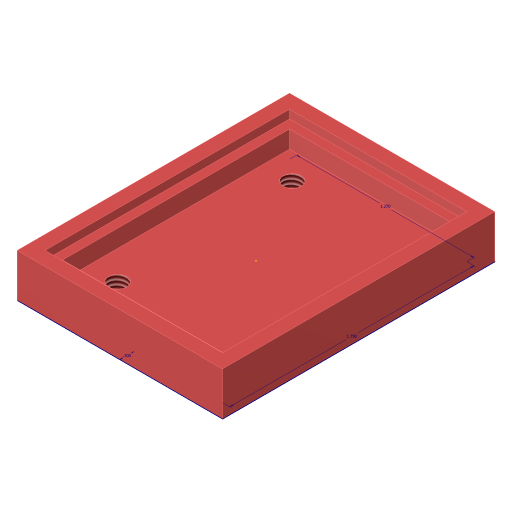
# Autodesk Inventor part: TOF mount
Saved by Autodesk Inventor 2023.4 (Build 274418000, 418)
## iProperties
Created: 2025-02-18
Part Number: TOF mount
Material: ABS Plastic
Document SubType Name: Modeling
Designer: mavericks
Density: 1.06 g/cm^3
Appearance: Smooth - Red
Author: mavericks
Autodesk Inventor part; units mm, degrees
ref_plane "YZ Plane" through (0, 0, 0) normal (1, 0, 0) x (0, 1, 0)
ref_plane "XZ Plane" through (0, 0, 0) normal (0, 1, 0) x (-1, 0, 0)
ref_plane "XY Plane" through (0, 0, 0) normal (0, 0, 1) x (1, 0, 0)
sketch "Sketch2" plane through (0, 0, 0) normal (0, 1, 0) x (-1, 0, 0)
  line L0 (16.129, 22.225) -> (-16.129, 22.225)
  line L1 (-16.129, 22.225) -> (-16.129, -22.225)
  line L2 (-16.129, -22.225) -> (16.129, -22.225)
  line L3 (16.129, -22.225) -> (16.129, 22.225)
  line L4 (16.129, 22.225) -> (-16.129, -22.225) construction
  line L5 (-16.129, 22.225) -> (16.129, -22.225) construction
  line L6 (-18.669, 24.765) -> (18.669, 24.765)
  line L7 (18.669, 24.765) -> (18.669, -24.765)
  line L8 (18.669, -24.765) -> (-18.669, -24.765)
  line L9 (-18.669, -24.765) -> (-18.669, 24.765)
  point P0 (0, 0)
  dimension "d0" = 32.258
  dimension "d1" = 44.45
  dimension "d2" = 2.54
  constraints: 20 end point, 4 parallel, 2 midpoint, 2 perpendicular, 1 horizontal, 3 other
  measures "d0" distance of L2.end L1.end
  measures "d1" distance of L1.end L0.end
  measures "d2" distance between parallel lines of L0 L6
extrude "Extrusion1" add sketch "Sketch2" along normal blind 3.175 contours L3 L2 L1 L0
extrude "Extrusion2" add sketch "Sketch2" along normal blind 7.874
sketch "Sketch3" plane through (0, 3.175, 0) normal (0, 1, 0) x (1, 0, 0)
  line L0 (16.129, 22.225) -> (16.129, -22.225) projected
  line L1 (16.129, -22.225) -> (-16.129, -22.225) projected
  point P0 (0, 0)
  point P1 (-9.271, -15.875)
  point P2 (-9.271, 15.875)
  dimension "d7" = 25.4
  dimension "d8" = 25.4
  dimension "d9" = 6.35
  dimension "d10" = 38.1
  measures "d7" distance from line of L0 point (-9.271, -15.875)
  measures "d8" distance from line of L0 point (-9.271, 15.875)
  measures "d9" distance from line of point (-9.271, -15.875) L1
  measures "d10" distance from line of point (-9.271, 15.875) L1
hole "Hole1" at (-9.271, 3.175, 15.875) at (-9.271, 3.175, -15.875) direction (0, -1, 0) diameter 3.302 end through all thread size "8-32 UNC" class "2B" standard "ANSI Unified Screw Threads"
sketch "Sketch5" plane through (0, 3.175, 0) normal (0, 1, 0) x (1, 0, 0)
  point P0 (0, 0)
sketch "Sketch6" plane through (0, 3.175, 0) normal (0, 1, 0) x (1, 0, 0)
  line L0 (16.129, -22.225) -> (16.129, 22.225) projected
  line L1 (16.129, -20.6375) -> (-14.5415, -20.6375)
  line L2 (-14.5415, -20.6375) -> (-14.5415, 20.6375)
  line L3 (-14.5415, 20.6375) -> (16.129, 20.6375)
  line L4 (-16.129, -22.225) -> (16.129, -22.225) projected
  line L5 (-16.129, 22.225) -> (-16.129, -22.225) projected
  line L6 (16.129, 22.225) -> (-16.129, 22.225) projected
  point P0 (0, 0)
  dimension "d23" = 1.5875
  dimension "d24" = 1.5875
  dimension "d25" = 1.5875
  constraints: 6 end point, 2 perpendicular, 2 point on line, 1 horizontal
  measures "d23" distance between parallel lines of L4 L1
  measures "d24" distance between parallel lines of L2 L5
  measures "d25" distance between parallel lines of L6 L3
extrude "Extrusion4" add sketch "Sketch6" along normal blind 3.175 contours L4 L5 L6 L0 L3 L2 L1
equation "\"d8\" = d7"
body "Solid1"
